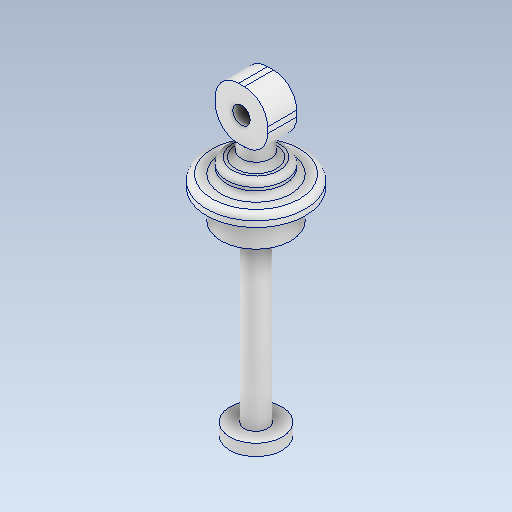
# Autodesk Inventor part: Tlok
Saved by Autodesk Inventor 2020.3 (Build 243373000, 373)
## iProperties
Created: 2021-03-25
Part Number: Tlok
Material: Aluminum 6061
Document SubType Name: Modeling
Designer: patry
Density: 2.7 g/cm^3
Appearance: Aluminum - Flat
Mass: 5.602 g
Surface Area: 16.3098 cm^2
Volume: 2.07482 cm^3
Author: patry
Autodesk Inventor part; units mm, degrees
ref_plane "YZ Plane" through (0, 0, 0) normal (1, 0, 0) x (0, 1, 0)
ref_plane "XZ Plane" through (0, 0, 0) normal (0, 1, 0) x (-1, 0, 0)
ref_plane "XY Plane" through (0, 0, 0) normal (0, 0, 1) x (1, 0, 0)
sketch "Szkic1" plane through (0, 0, 0) normal (0, 1, 0) x (-1, 0, 0)
  circle A0 centre (0, 0) radius 4.5
  dimension "d0" = 9
  constraints: 1 centre point, 1 coincident
  measures "d0" diameter of A0
extrude "Wyciągnięcie proste1" add sketch "Szkic1" along normal blind 2
sketch "Szkic2" plane through (0, 2, 0) normal (0, 1, 0) x (1, 0, 0)
  circle A0 centre (0, 0) radius 2
  dimension "d3" = 4
  constraints: 1 centre point, 1 coincident
  measures "d3" diameter of A0
extrude "Wyciągnięcie proste2" add sketch "Szkic2" along normal blind 30
sketch "Szkic3" plane through (0, 32, 0) normal (0, 1, 0) x (1, 0, 0)
  circle A0 centre (0, 0) radius 6
  dimension "d6" = 12
  constraints: 1 centre point, 1 coincident
  measures "d6" diameter of A0
extrude "Wyciągnięcie proste3" add sketch "Szkic3" along normal blind 5
sketch "Szkic4" plane through (0, 37, 0) normal (0, 1, 0) x (1, 0, 0)
  circle A0 centre (0, 0) radius 8.5
  dimension "d9" = 17
  constraints: 1 centre point, 1 coincident
  measures "d9" diameter of A0
extrude "Wyciągnięcie proste4" add sketch "Szkic4" along normal blind 2
sketch "Szkic5" plane through (0, 39, 0) normal (0, 1, 0) x (1, 0, 0)
  circle A0 centre (0, 0) radius 5
  dimension "d12" = 10
  constraints: 1 centre point, 1 coincident
  measures "d12" diameter of A0
extrude "Wyciągnięcie proste5" add sketch "Szkic5" along normal blind 2.5
sketch "Szkic6" plane through (0, 41.5, 0) normal (0, 1, 0) x (1, 0, 0)
  circle A0 centre (0, 0) radius 2.5
  dimension "d15" = 5
  constraints: 1 centre point, 1 coincident
  measures "d15" diameter of A0
extrude "Wyciągnięcie proste6" add sketch "Szkic6" along normal blind 3
sketch "Szkic7" plane through (0, 44.5, 0) normal (0, 1, 0) x (1, 0, 0)
  line L0 (4.5, -2.5) -> (-4.5, -2.5)
  line L1 (-4.5, -2.5) -> (-4.5, 2.5)
  line L2 (-4.5, 2.5) -> (4.5, 2.5)
  line L3 (4.5, 2.5) -> (4.5, -2.5)
  line L4 (4.5, -2.5) -> (-4.5, 2.5) construction
  line L5 (-4.5, -2.5) -> (4.5, 2.5) construction
  point P0 (0, 0)
  dimension "d18" = 9
  dimension "d19" = 5
  constraints: 12 end point, 2 midpoint, 2 parallel, 1 horizontal, 1 perpendicular
  measures "d18" distance of L1.end L2.end
  measures "d19" distance of L0.end L1.end
extrude "Wyciągnięcie proste7" add sketch "Szkic7" along normal blind 9
fillet "Zaokrąglenie1" radius 4 4 edges at (4.5, 44.5, 0) (4.5, 53.5, 0) (-4.5, 53.5, 0) (-4.5, 44.5, 0)
sketch "Szkic8" plane through (-0.5, 44.5, 2.5) normal (0, 0, 1) x (1, 0, 0)
  line L0 (0, 9) -> (1, 9) projected
  line L1 (-4, 4) -> (-4, 5) projected
  circle A0 centre (0.5, 4.5) radius 1.5
  line L2 (0, 0) -> (0.5, 0) projected
  line L3 (5, 4) -> (5, 5) projected
  point P0 (0.5, -44.5)
  dimension "d23" = 3
  dimension "d26" = 9
  dimension "d27" = 9
  dimension "d28" = 4.5
  dimension "d29" = 4.5
  constraints: 1 centre point, 1 coincident
  measures "d23" diameter of A0
  measures "d26" distance between parallel lines of L2 L0
  measures "d27" distance between parallel lines of L3 L1
  measures "d28" distance from line of L0 A0.centre
  measures "d29" distance from line of L1 point (0.5, 4.5)
extrude "Wyciągnięcie proste8" cut sketch "Szkic8" against normal blind 10
fillet "Zaokrąglenie2" radius 1 4 edges at (-8.5, 39, 0) (-5, 39, 0) (-5, 41.5, 0) (-2.5, 41.5, 0)
equation "\"d28\" = 0.5 * d26"
equation "\"d29\" = 0.5 * d27"
